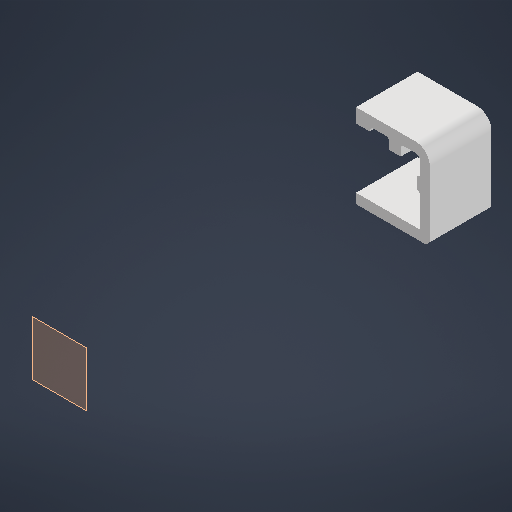
# Autodesk Inventor part: HangerNinety
Saved by Autodesk Inventor 2026.1 (Build 301233020, 233B)
## iProperties
Created: 2025-09-15
Part Number: HangerNinety
Material: Generic
Document SubType Name: Modeling
Designer: atrus
Density: 1 g/cm^3
Appearance: Default
Author: atrus
Autodesk Inventor part; units mm, degrees
ref_plane "YZ Plane" through (0, 0, 0) normal (1, 0, 0) x (0, 1, 0)
ref_plane "XZ Plane" through (0, 0, 0) normal (0, 1, 0) x (-1, 0, 0)
ref_plane "XY Plane" through (0, 0, 0) normal (0, 0, 1) x (1, 0, 0)
ref_plane "Work Plane2" through (0, 0, -200) normal (0, 0, 1) x (1, 0, 0)
ref_plane "Work Plane1" through (0, 0, 0) normal (0, 0, 1) x (1, 0, 0)
sketch "Sketch1" plane through (0, 0, -200) normal (0, 0, 1) x (1, 0, 0)
  arc A0 (6.1983, 20.8783) -> (6.1983, 23.0183) centre (6.1983, 21.9483) ccw construction
  line L0 (12.2867, 14.8983) -> (8.7499, 14.8983) construction
  arc A1 (14.8383, 23.0183) -> (14.8383, 20.8783) centre (14.8383, 21.9483) ccw construction
  arc A2 (23.0183, 21.0366) -> (21.0366, 23.0183) centre (21.0366, 21.0366) ccw construction
  line L1 (21.0366, 23.0183) -> (14.8383, 23.0183) construction
  arc A3 (20.8783, 14.8383) -> (23.0183, 14.8383) centre (21.9483, 14.8383) ccw construction
  line L2 (23.0183, 14.8383) -> (23.0183, 21.0366) construction
  line L3 (14.8983, 8.7499) -> (14.8983, 12.2867) construction
  line L4 (-1.9817, 21.0366) -> (-1.9817, 0) construction
  arc A4 (-1.9817, 0) -> (0, -1.9817) centre (0, 0) ccw construction
  line L5 (0, -1.9817) -> (6.1983, -1.9817) construction
  line L6 (14.8383, -1.9817) -> (21.0366, -1.9817) construction
  arc A5 (21.0366, -1.9817) -> (23.0183, 0) centre (21.0366, 0) ccw construction
  line L7 (23.0183, 0) -> (23.0183, 6.1983) construction
  arc A6 (23.0183, 6.1983) -> (20.8783, 6.1983) centre (21.9483, 6.1983) ccw construction
  line L8 (20.8783, 6.1983) -> (20.8783, 4.0901) construction
  arc A7 (19.1681, 3.3817) -> (20.8783, 4.0901) centre (19.8765, 4.0901) ccw construction
  line L9 (19.1681, 3.3817) -> (15.675, 6.8748) construction
  arc A8 (14.8983, 8.7499) -> (15.675, 6.8748) centre (17.55, 8.7499) ccw construction
  line L10 (15.675, 14.1617) -> (19.1681, 17.6549) construction
  arc A9 (15.675, 14.1617) -> (14.8983, 12.2867) centre (17.55, 12.2867) ccw construction
  line L11 (20.8783, 16.9465) -> (20.8783, 14.8383) construction
  arc A10 (20.8783, 16.9465) -> (19.1681, 17.6549) centre (19.8765, 16.9465) ccw construction
  line L12 (17.6549, 19.1681) -> (14.1617, 15.675) construction
  arc A11 (17.6549, 19.1681) -> (16.9465, 20.8783) centre (16.9465, 19.8765) ccw construction
  line L13 (14.8383, 20.8783) -> (16.9465, 20.8783) construction
  arc A12 (12.2867, 14.8983) -> (14.1617, 15.675) centre (12.2867, 17.55) ccw construction
  arc A13 (6.8748, 15.675) -> (8.7499, 14.8983) centre (8.7499, 17.55) ccw construction
  line L14 (6.8748, 15.675) -> (3.3817, 19.1681) construction
  arc A14 (4.0901, 20.8783) -> (3.3817, 19.1681) centre (4.0901, 19.8765) ccw construction
  line L15 (4.0901, 20.8783) -> (6.1983, 20.8783) construction
  line L16 (6.1983, 23.0183) -> (0, 23.0183) construction
  arc A15 (0, 23.0183) -> (-1.9817, 21.0366) centre (0, 21.0366) ccw construction
  line L17 (7.4683, 21.9483) -> (7.4683, 17.8983)
  line L18 (7.4683, 17.8983) -> (13.5683, 17.8983)
  line L19 (13.5683, 17.8983) -> (13.5683, 21.9483)
  arc A16 (7.4683, 21.9483) -> (6.1983, 23.2183) centre (6.1983, 21.9483) ccw
  arc A17 (14.8383, 23.2183) -> (13.5683, 21.9483) centre (14.8383, 21.9483) ccw
  line L20 (6.1983, 23.2183) -> (0, 23.2183)
  line L21 (0, 23.2183) -> (0, 28.2183)
  line L22 (0, 28.2183) -> (21.0366, 28.2183)
  arc A18 (23.2183, 21.0366) -> (21.0366, 23.2183) centre (21.0366, 21.0366) ccw
  line L23 (23.2183, 21.0366) -> (23.2183, 14.8383)
  arc A19 (21.9483, 13.5683) -> (23.2183, 14.8383) centre (21.9483, 14.8383) ccw
  arc A20 (28.2183, 21.0366) -> (21.0366, 28.2183) centre (21.0366, 21.0366) ccw
  line L24 (28.2183, 21.0366) -> (28.2183, 0)
  line L25 (21.9483, 13.5683) -> (21.9483, 7.4683)
  arc A21 (23.2183, 6.1983) -> (21.9483, 7.4683) centre (21.9483, 6.1983) ccw
  line L26 (23.2183, 6.1983) -> (23.2183, -8.9287)
  line L27 (23.0183, -9.1287) -> (-9, -9.1287)
  line L28 (-9, -9.1287) -> (-9, -14.1287)
  line L29 (-9, -14.1287) -> (26.2183, -14.1287)
  line L30 (28.2183, -12.1287) -> (28.2183, 0)
  arc A22 (23.0183, -9.1287) -> (23.2183, -8.9287) centre (23.0183, -8.9287) ccw
  line L31 (14.8383, 23.2183) -> (21.0366, 23.2183)
  line L32 (0, 28.2183) -> (-9, 28.2183)
  arc A23 (0, 23.2183) -> (-2.1817, 21.0366) centre (0, 21.0366) ccw
  line L33 (-2.1817, 21.0366) -> (-9, 21.0366)
  line L34 (-9, 21.0366) -> (-9, 28.2183)
  circle A24 centre (-5.5909, 22.0366) radius 2
  line L35 (-5.5909, 21.0366) -> (-5.5909, 28.2183) construction
  line L36 (-5.5909, 21.0366) -> (-5.5909, -14.1287) construction
  circle A25 centre (-5.5909, -10.1287) radius 2
  line L37 (26.2183, -14.1287) -> (28.2183, -12.1287)
  point P0 (0, 0)
  point P1 (7.2683, 21.9483)
  point P2 (10.5183, 14.8983)
  point P3 (10.5183, 17.8983)
  point P4 (13.7683, 21.9483)
  point P5 (23.0183, -8.9287)
  point P6 (-1.9817, -8.9287)
  point P7 (28.2183, -14.1287)
  point P8 (17.4722, 23.2183)
  point P9 (-9, 24.6274)
  point P10 (-3.8588, -9.1287)
  point P11 (-7.3229, -9.1287)
  point P12 (-7.3229, 21.0366)
  point P13 (-3.8588, 21.0366)
  dimension "d1" = 0.2
  dimension "d2" = 3
  dimension "d3" = 0.2
  dimension "d4" = 0.2
  dimension "d5" = 0.2
  dimension "d6" = 5
  dimension "d7" = 5
  dimension "d8" = 5
  dimension "d9" = 0.2
  dimension "d13" = 9
  dimension "d14" = 4
  dimension "d15" = 1
  dimension "d16" = 4
  dimension "d17" = 1
  dimension "d18" = 135
  dimension "d19" = 2
  constraints: 42 end point, 18 point on circle, 10 centre point, 8 horizontal alignment, 8 perpendicular, 8 vertical, 8 vertical alignment, 7 coincident, 6 point on line, 4 midpoint, 3 horizontal, 2 tangent, 1 collinear, 2 other
  measures "d1" distance from line of L17 point (7.268, 21.948)
  measures "d2" distance of point (10.518, 14.898) point (10.518, 17.898)
  measures "d3" distance between parallel lines of L23 L2
  measures "d4" distance of L26.start L7.end
  measures "d5" radius of A22
  measures "d6" distance between parallel lines of L30 L26
  measures "d7" distance between parallel lines of L27 L29
  measures "d8" distance from line of L22 point (17.472, 23.218)
  measures "d9" distance from line of point (23.018, -8.929) L27
  measures "d13" distance from line of L21 point (-9, 24.627)
  measures "d14" diameter of A24
  measures "d15" distance of L35.start A24.centre
  measures "d16" diameter of A25
  measures "d17" distance from line of L27 A25.centre
  measures "d18" angle of L37 L30
  measures "d19" horizontal distance of L29.end L30.start
extrude "Extrusion1" add sketch "Sketch1" along normal blind 31 contours A16 L20 L21 L22 A20 L24 L30 L37 L29 L28 L27 A25 A22 L26 A21 L25 A19 L23 A18 L31 A17 L19 L18 L17 | A23 L33 A24 L34 L32 L21 | L33 A24 | L27 A25 picked at (-4.9344, 21.2542) picked at (-5.9682, -10.8067)
body "Solid1"
